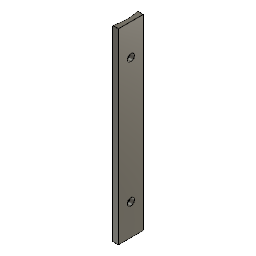
Pre+Filter+Sheet (Autodesk Fusion 360 design; units mm, degrees)
Autodesk Fusion 360 part; units mm, degrees
sketch "Sketch1" plane through (0, 0, 0) normal (0, 0, 1) x (1, 0, 0)
  circle A0 centre (0, 0) radius 22.5
  circle A1 centre (10.9935, 0) radius 15
  line L0 (21.0297, 6) -> (24.7412, 6)
  line L1 (21.3005, -6) -> (24.7412, -6)
  line L2 (-24.0211, 0.3833) -> (-31.0114, 0.3928) construction
  line L3 (0, 0) -> (31, 0) construction
  dimension "d2" = 45
  dimension "d3" = 30
  dimension "d6" = 6
  dimension "d7" = 6
  constraint horizontal A0.centre A1.centre
  constraint coincident A1 L0.end
  constraint horizontal L0
  constraint coincident A1 L1.end
  constraint parallel L0 L1
  constraint coincident A0.centre L3.start
  constraint horizontal L3
  constraint coincident A1.centre L3
  measures "d2" diameter of A0
  measures "d3" diameter of A1
  measures "d6" distance of L1 L3
  measures "d7" distance of L0 L3
extrude "Extrude1" add sketch "Sketch1" along normal blind 90 contours A0 A1 L0 L1
ref_plane "WorkPlane1" through (25.9935, 0, 55.0321) normal (1, 0, 0) x (0, -1, 0)
sketch "Sketch2" plane through (25.9935, 0, 0) normal (1, 0, 0) x (0, 1, 0)
  circle A0 centre (0, 75) radius 1.7
  circle A1 centre (0, 15) radius 1.7
  line L0 (6, 90) -> (-6, 90)
  dimension "d11" = 60
  dimension "d12" = 3.4
  dimension "d15" = 15
  constraint equal A0 A1
  measures "d11" distance of A0.centre A1.centre
  measures "d12" diameter of A0
  measures "d15" distance of A0.centre L0
extrude "Extrude2" cut sketch "Sketch2" against normal blind 25
ref_plane "WorkPlane2" through (25.9935, 0, 73.0088) normal (1, 0, 0) x (0, -1, 0)
sketch "Sketch3" plane through (25.9935, 0, 0) normal (1, 0, 0) x (0, 1, 0)
  line L0 (-6, 90) -> (6, 90)
  line L1 (6, 90) -> (6, 0)
  line L2 (6, 0) -> (-6, 0)
  line L3 (-6, 0) -> (-6, 90)
  line L4 (0, 0) -> (0, 98.2362) construction
  dimension "d22" = 12
  dimension "d23" = 6
  constraint horizontal L0
  constraint vertical L1
  constraint horizontal L2
  constraint vertical L3
  constraint coincident L4.start origin
  constraint perpendicular L0 L4
  measures "d22" distance of L0.start L0.end
  measures "d23" distance of L3 L4
extrude "Extrude3" cut sketch "Sketch3" against normal blind 1.5
